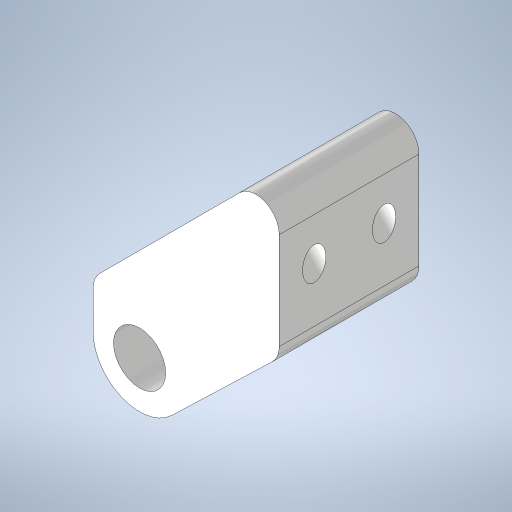
# Autodesk Inventor part: Wedge Mount
Saved by Autodesk Inventor 2023.2 (Build 272271000, 271)
## iProperties
Created: 2024-04-01
Part Number: Wedge Mount
Material: UHMW, White
Document SubType Name: Modeling
Designer: Nathan Cai
Density: 0.94 g/cm^3
Appearance: Smooth - White
Mass: 7.49207 g
Surface Area: 37.8303 cm^2
Volume: 7.97029 cm^3
Author: Nathan Cai
Autodesk Inventor part; units mm, degrees
ref_plane "YZ Plane" through (0, 0, 0) normal (1, 0, 0) x (0, 1, 0)
ref_plane "XZ Plane" through (0, 0, 0) normal (0, 1, 0) x (-1, 0, 0)
ref_plane "XY Plane" through (0, 0, 0) normal (0, 0, 1) x (1, 0, 0)
sketch "Sketch1" plane through (0, 0, 0) normal (0, 0, 1) x (1, 0, 0)
  circle A0 centre (0, 0) radius 3.556
  circle A1 centre (0, 0) radius 6.35
  line L0 (-6.35, 0) -> (-6.35, 6.35)
  line L1 (-6.35, 6.35) -> (19.05, 31.75)
  line L2 (19.05, 31.75) -> (19.05, 9.525)
  line L3 (19.05, 9.525) -> (4.404, -4.5746)
  dimension "d0" = 7.112
  dimension "d1" = 12.7
  dimension "d2" = 45
  dimension "d4" = 25.4
  dimension "d5" = 31.75
  dimension "d6" = 9.525
  constraints: 8 end point, 2 centre point, 2 coincident, 2 point on circle, 2 tangent, 2 vertical
  measures "d0" diameter of A0
  measures "d1" diameter of A1
  measures "d2" angle of L2 L1
  measures "d4" distance between parallel lines of L0 L2
  measures "d5" vertical distance of A1.centre L1.end
  measures "d6" vertical distance of A1.centre L2.end
extrude "Extrusion1" add sketch "Sketch1" along normal blind 19.05
sketch "Sketch2" plane through (-6.35, 6.35, 0) normal (-0.7071068, 0.7071068, 0) x (-0.7071068, -0.7071068, 0)
  line L0 (0, 0) -> (0, 19.05) projected
  line L1 (0, 9.525) -> (-35.921, 9.525) construction
  line L2 (-35.921, 0) -> (-35.921, 19.05) projected
  circle A0 centre (-26.396, 4.7625) radius 1.5875
  circle A1 centre (-26.396, 14.2875) radius 1.5875
  circle A2 centre (-16.871, 4.7625) radius 1.5875
  circle A3 centre (-16.871, 14.2875) radius 1.5875
  circle A4 centre (-7.346, 4.7625) radius 1.5875
  circle A5 centre (-7.346, 14.2875) radius 1.5875
  point P0 (-17.9605, 9.525)
  dimension "d9" = 3.175
  dimension "d10" = 4.7625
  dimension "d11" = 9.525
  dimension "d14" = 9.525
  dimension "d17" = 9.525
  constraints: 6 centre point, 3 midpoint, 2 end point, 1 horizontal, 1 vertical, 10 other
  measures "d9" diameter of A0
  measures "d10" vertical distance of point (-17.961, 9.525) A0.centre
  measures "d11" distance from line of L2 A0.centre
  measures "d14" distance of A0.centre A1.centre
  measures "d17" distance of A0.centre A2.centre
extrude "Extrusion2" cut sketch "Sketch2" against normal through all
fillet "Fillet1" radius 3.175 3 edges at (19.05, 31.75, 9.525) (19.05, 9.525, 9.525) (-6.35, 6.35, 9.525)
body "Solid1"
